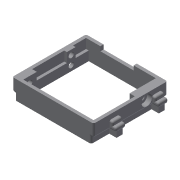
# Autodesk Inventor part: HDB Support
Saved by Autodesk Inventor 2017 (Build 210142000, 142)
## iProperties
Created: 2015-03-18
Part Number: HDB Support
Material: Generic
Document SubType Name: Modeling
Designer: PC-fabtotum
Density: 1 g/cm^3
Appearance: Default
RuleStatus: InUse
BeforeDocSave0: Spessore
Author: PC-fabtotum
Autodesk Inventor part; units mm, degrees
note: some values were not read from the file. Chosen so that the rebuilt part matches the saved one: second side of "Extrusion1".
ref_plane "Work Plane1" through (0, 0, -8.25) normal (0, 0, 1) x (1, 0, 0)
sketch "Sketch1" plane through (0, 0, -8.25) normal (0, 0, 1) x (1, 0, 0)
  line L0 (-37.1615, 17.9395) -> (9.3315, 17.9395)
  line L1 (9.3315, 17.9395) -> (9.3315, -24.2572)
  line L2 (9.3315, -24.2572) -> (-37.1615, -24.2572)
  line L3 (-37.1615, -24.2572) -> (-37.1615, 17.9395)
  point P0 (0, 0)
  constraints: 8 end point, 3 horizontal, 2 parallel, 2 vertical, 1 perpendicular, 1 other
extrude "Extrusion1" add sketch "Sketch1" along normal blind 7.25
sketch "Sketch2" plane through (0, 0, -8.25) normal (0, 0, 1) x (1, 0, 0)
  line L0 (13.1261, 14.7262) -> (3.5753, 14.7262)
  line L1 (3.5753, 14.7262) -> (3.5753, 9.2758)
  line L2 (3.5753, 9.2758) -> (13.1261, 9.2758)
  line L3 (13.1261, 9.2758) -> (13.1261, 14.7262)
  line L4 (13.1261, -9.4662) -> (3.7861, -9.4662)
  line L5 (3.7861, -9.4662) -> (3.7861, -15.116)
  line L6 (3.7861, -15.116) -> (13.1261, -15.116)
  line L7 (13.1261, -15.116) -> (13.1261, -9.4662)
  line L8 (-40.7637, 14.7262) -> (-33.7354, 14.7262)
  line L9 (-33.7354, 14.7262) -> (-33.7354, 9.2758)
  line L10 (-33.7354, 9.2758) -> (-40.7637, 9.2758)
  line L11 (-40.7637, 9.2758) -> (-40.7637, 14.7262)
  line L12 (-40.7637, -9.3156) -> (-33.2967, -9.3156)
  line L13 (-33.2967, -9.3156) -> (-33.2967, -15.116)
  line L14 (-33.2967, -15.116) -> (-40.7637, -15.116)
  line L15 (-40.7637, -15.116) -> (-40.7637, -9.3156)
  point P0 (0, 0)
  constraints: 32 end point, 11 horizontal, 8 parallel, 8 vertical, 5 point on line, 4 perpendicular, 17 other
extrude "Extrusion2" add sketch "Sketch2" along normal blind 2.5
sketch "Sketch3" plane through (0, 0, -5.75) normal (0, 0, 1) x (1, 0, 0)
  line L0 (9.3315, 9.2758) -> (13.1261, 9.2758) projected
  line L1 (11.304, 9.2758) -> (9.3315, 9.2758)
  line L2 (9.3315, 9.2758) -> (9.3315, 14.7262)
  line L3 (9.3315, 14.7262) -> (11.304, 14.7262)
  line L4 (11.304, 14.7262) -> (11.304, 9.2758)
  line L5 (9.3315, -24.2572) -> (9.3315, 17.9395) projected
  line L6 (13.1261, -9.4662) -> (9.3315, -9.4662) projected
  line L7 (11.304, -9.4662) -> (9.3315, -9.4662)
  line L8 (9.3315, -9.4662) -> (9.3315, -15.116)
  line L9 (9.3315, -15.116) -> (11.304, -15.116)
  line L10 (11.304, -15.116) -> (11.304, -9.4662)
  line L11 (-37.1615, -15.116) -> (-38.9272, -15.116)
  line L12 (-38.9272, -15.116) -> (-38.9272, -9.3156)
  line L13 (-38.9272, -9.3156) -> (-37.1615, -9.3156)
  line L14 (-37.1615, -9.3156) -> (-37.1615, -15.116)
  line L15 (-37.1615, 14.7262) -> (-40.7637, 14.7262) projected
  line L16 (-38.9272, 14.7262) -> (-37.1615, 14.7262)
  line L17 (-37.1615, 14.7262) -> (-37.1615, 9.2758)
  line L18 (-37.1615, 9.2758) -> (-38.9272, 9.2758)
  line L19 (-38.9272, 9.2758) -> (-38.9272, 14.7262)
  line L20 (13.1261, 14.7262) -> (9.3315, 14.7262) projected
  line L21 (-37.1615, -9.3156) -> (-40.7637, -9.3156) projected
  point P0 (0, 0)
  constraints: 32 end point, 8 parallel, 5 collinear, 4 horizontal, 4 perpendicular, 3 point on line, 2 vertical
extrude "Extrusion3" add sketch "Sketch3" along normal blind 2
sketch "Sketch4" plane through (0, 0, -8.25) normal (0, 0, -1) x (-1, 0, 0)
  line L0 (-9.3315, -24.2572) -> (37.1615, -24.2572) projected
  line L1 (37.1615, 17.9395) -> (-9.3315, 17.9395) projected
  line L2 (-7.9441, -24.2572) -> (35.6472, -24.2572)
  line L3 (35.6472, -24.2572) -> (35.6472, 17.9395)
  line L4 (35.6472, 17.9395) -> (-7.9441, 17.9395)
  line L5 (-7.9441, 17.9395) -> (-7.9441, -24.2572)
  point P0 (0, 0)
  constraints: 8 end point, 2 parallel, 2 point on line, 1 horizontal, 1 perpendicular
extrude "Extrusion4" add sketch "Sketch4" along normal blind 3.5
shell "Shell1" thickness 1.8 removed faces 1 at (-21.6638, -10.1916, -1)
sketch "Sketch5" plane through (-33.8472, -22.4572, -9.95) normal (0, 0, 1) x (1, 0, 0)
  line L0 (41.3787, 38.5966) -> (41.3787, 0) construction
  line L1 (41.3787, 23.5966) -> (38.3787, 23.5966)
  line L2 (38.3787, 23.5966) -> (38.3787, 38.5966)
  line L3 (38.3787, 38.5966) -> (41.3787, 38.5966)
  line L4 (41.3787, 23.5966) -> (41.3787, 38.5966)
  line L5 (-1.8, -1.0089) -> (1.1787, -1.0089)
  line L6 (1.1787, -1.0089) -> (1.1787, 7.7162)
  line L7 (1.1787, 7.7162) -> (-1.8, 7.7162)
  line L8 (-1.8, 7.7162) -> (-1.8, -1.0089)
  line L9 (-1.8, -1.8) -> (-1.8, 40.3966) projected
  line L10 (0, 0) -> (0, 38.5966) projected
  line L11 (41.3787, 33.5329) -> (41.3787, 11.191) projected
  line L12 (0, 38.5966) -> (39.9913, 38.5966) projected
  point P0 (33.8472, 22.4572)
  dimension "d69" = 37.2
  dimension "d70" = 3
  dimension "d71" = 15
  constraints: 16 end point, 3 collinear, 3 perpendicular, 2 horizontal, 2 parallel, 2 point on line
  measures "d69" distance between parallel lines of L6 L2
  measures "d70" distance between parallel lines of L2 L11
  measures "d71" distance of L1.end L2.end
extrude "Extrusion5" add sketch "Sketch5" along normal up to surface (8.95 mm away)
sketch "Sketch6" plane through (-37.1615, -24.2572, -1) normal (-1, 0, 0) x (0, 0, 1)
  point P0 (1, 24.2572)
  point P1 (-3.6337, 5.4847)
hole "Hole1" at (-37.1615, -18.7725, -4.6337) direction (1, 0, 0) diameter 3 depth 8 tip angle 118 counterbore diameter 6 counterbore depth 2.7
sketch "Sketch7" plane through (9.3315, -24.2572, -1) normal (1, 0, 0) x (0, 0, -1)
  point P0 (-1, 24.2572)
  point P1 (3.6353, 30.4382)
hole "Hole2" at (9.3315, 6.181, -4.6353) direction (-1, 0, 0) diameter 3 depth 8 tip angle 118 counterbore diameter 6 counterbore depth 2.7
sketch "Sketch8" plane through (-33.8472, 16.1395, -9.95) normal (0, 0, 1) x (1, 0, 0)
  line L0 (1.1787, -38.5966) -> (3.957, -38.5966)
  line L1 (3.957, -38.5966) -> (3.957, -39.3714)
  line L2 (3.957, -39.3714) -> (1.1787, -39.3714)
  line L3 (1.1787, -39.3714) -> (1.1787, -38.5966)
  circle A0 centre (30.4917, -32.0966) radius 7.5
  line L4 (30.4917, -32.0966) -> (30.4917, -39.5966) construction
  line L5 (-3.3143, -40.3966) -> (43.1787, -40.3966) projected
  line L6 (39.9913, -38.5966) -> (39.9913, -15) projected
  point P0 (33.8472, -16.1395)
  dimension "d51" = 15
  dimension "d50" = 0.8
  dimension "d52" = 9.4996
  constraints: 10 end point, 2 parallel, 1 horizontal, 1 perpendicular, 1 vertical, 1 vertical alignment, 2 other
  measures "d50" distance from line of L5 L4.end
  measures "d52" distance between parallel lines of L6 L4
extrude "Extrusion6" [suppressed]
sketch "Sketch9" plane through (-33.8472, 16.1395, -9.95) normal (0, 0, 1) x (1, 0, 0)
  line L0 (39.9913, -38.5966) -> (1.1787, -38.5966) construction
  line L1 (6.3811, -38.5966) -> (19.879, -38.5966)
  line L2 (19.879, -38.5966) -> (19.879, -22.0157)
  line L3 (19.879, -22.0157) -> (6.3811, -22.0157)
  line L4 (6.3811, -22.0157) -> (6.3811, -38.5966)
  line L5 (0, 0) -> (38.3787, 0) construction
  line L6 (33.1556, 0) -> (28.7955, 0)
  line L7 (28.7955, 0) -> (28.7955, -12.1404)
  line L8 (28.7955, -12.1404) -> (33.1556, -12.1404)
  line L9 (33.1556, -12.1404) -> (33.1556, 0)
  point P0 (33.8472, -16.1395)
  point P1 (26.0223, -38.1966)
  point P2 (3.6113, -38.1966)
  point P3 (39.9913, 0)
  constraints: 16 end point, 4 parallel, 2 horizontal, 2 perpendicular, 1 point on line, 2 other
extrude "Extrusion7" [suppressed]
sketch "Sketch10" plane through (-33.8472, -14.741, -9.95) normal (0, 0, 1) x (1, 0, 0)
  arc A0 (2.5514, 21.9404) -> (28.5514, 21.9404) centre (15.5514, 21.9404) ccw
  line L0 (28.5514, 21.9404) -> (28.5514, 32.6805)
  line L1 (28.5514, 32.6805) -> (2.5514, 32.6805)
  line L2 (2.5514, 32.6805) -> (2.5514, 21.9404)
  line L3 (43.1787, 32.6805) -> (-3.3143, 32.6805) projected
  line L4 (15.5514, 21.9404) -> (15.5514, 32.6805)
  line L5 (-1.8, 32.6805) -> (41.7913, 32.6805) projected
  line L6 (0, 30.8805) -> (0, 0) projected
  point P0 (33.8472, 14.741)
  dimension "d32" = 13
  dimension "d53" = 10.7401
  dimension "d54" = 15.5513
  constraints: 8 end point, 2 point on circle, 2 tangent, 1 centre point, 1 collinear, 1 parallel, 1 perpendicular, 1 point on line, 1 vertical
  measures "d32" radius of A0
  measures "d53" distance of L4.start L4.end
  measures "d54" distance between parallel lines of L6 L4
extrude "Extrusion8" [suppressed]
shell "Shell2" [suppressed]
fillet "Fillet1" [suppressed]
fillet "Fillet3" radius 1 70 edges at (-39.8455, -15.116, -5.75) (-40.7637, -15.116, -7) (-40.7637, -12.2158, -5.75) (-39.8455, -9.3156, -5.75) (-40.7637, -9.3156, -7) (-38.9272, -15.116, -4.75) (-38.9272, -9.3156, -4.75) (-38.9272, -12.2158, -3.75) (-38.0444, -9.3156, -3.75) (-38.0444, -15.116, -3.75) (-38.9626, -15.116, -8.25) (-40.7637, -12.2158, -8.25) (-38.9626, -9.3156, -8.25) (-37.1615, -19.6866, -8.25) (-36.4043, -24.2572, -8.25) (-35.6472, -24.2572, -10) (-37.1615, -24.2572, -4.625) (-40.7637, 9.2758, -7) (-39.8455, 9.2758, -5.75) (-39.8455, 14.7262, -5.75) (-40.7637, 12.001, -5.75) (-40.7637, 14.7262, -7) (-40.7637, 12.001, -8.25) (-38.9626, 9.2758, -8.25) (-38.9626, 14.7262, -8.25) (-38.9272, 14.7262, -4.75) (-38.9272, 9.2758, -4.75) (-38.0444, 9.2758, -3.75) (-38.9272, 12.001, -3.75) (-38.0444, 14.7262, -3.75) (-37.1615, -0.0199, -8.25) (-37.1615, 16.3328, -8.25) (-37.1615, 17.9395, -4.625) (-35.6472, 17.9395, -10) (-36.4043, 17.9395, -8.25) (13.1261, -12.2911, -8.25) (11.2288, -15.116, -8.25) (13.1261, -15.116, -7) (13.1261, -9.4662, -7) (13.1261, -12.2911, -5.75) (12.215, -9.4662, -5.75) (12.215, -15.116, -5.75) (10.3178, -15.116, -3.75) (11.304, -12.2911, -3.75) (11.304, -15.116, -4.75) (11.304, -9.4662, -4.75) (10.3178, -9.4662, -3.75) (9.3315, -19.6866, -8.25) (9.3315, -0.0952, -8.25) (7.9441, -24.2572, -10) (8.6378, -24.2572, -8.25) (9.3315, -24.2572, -4.625) (13.1261, 14.7262, -7) (13.1261, 9.2758, -7) (13.1261, 12.001, -5.75) (12.215, 14.7262, -5.75) (12.215, 9.2758, -5.75) (13.1261, 12.001, -8.25) (11.2288, 14.7262, -8.25) (11.2288, 9.2758, -8.25) (11.304, 9.2758, -4.75) (11.304, 12.001, -3.75) (10.3178, 9.2758, -3.75) (10.3178, 14.7262, -3.75) (11.304, 14.7262, -4.75) (9.3315, 16.3328, -8.25) (8.6378, 17.9395, -8.25) (9.3315, 17.9395, -4.625) (7.9441, 17.9395, -10) (11.2288, -9.4662, -8.25)
sketch "Sketch12" plane through (0, 0, -11.75) normal (0, 0, -1) x (-1, 0, 0)
  circle A0 centre (3.536, -9.9787) radius 7.2457
  point P0 (0, 0)
  constraints: 1 centre point
extrude "Extrusion9" [suppressed]
fillet "Fillet4" radius 0.5 3 edges at (-35.3543, -23.9643, -7.9571) (-35.3543, 17.6466, -7.9571) (-35.6472, -3.1588, -8.25)
sketch "Sketch13" plane through (0, 0, -8.25) normal (0, 0, -1) x (-1, 0, 0)
  line L0 (-12.1261, 13.7262) -> (-12.1261, 10.2758)
  line L1 (-12.1261, 13.7262) -> (-12.1261, 10.2758) projected
  line L2 (-12.1261, 10.2758) -> (-7.9441, 10.2758)
  line L3 (-12.1261, 13.7262) -> (-7.9441, 13.7262)
  line L4 (-7.9441, 13.2762) -> (-11.6761, 13.2762)
  line L5 (-11.6761, 13.2762) -> (-11.6761, 10.7258)
  line L6 (-11.6761, 10.7258) -> (-7.9441, 10.7258)
  line L7 (-7.9441, 13.7262) -> (-7.9441, 13.2762)
  line L8 (-7.9441, -23.2572) -> (-7.9441, 16.9395) projected
  line L9 (-7.9441, 10.7258) -> (-7.9441, 10.2758)
  point P0 (0, 0)
  dimension "d46" = 0.45
  constraints: 16 end point, 3 collinear, 2 parallel, 2 perpendicular, 2 other
  measures "d46" distance between parallel lines of L2 L6
extrude "Extrusion10" add sketch "Sketch13" along normal up to surface (3.5 mm away) contours L3 L7 L4 L5 L6 L8 L2 L0
ref_plane "Work Plane2" through (9.3315, -0.0952, -7.25) normal (0, 1, 0) x (1, 0, 0)
ref_plane "Work Plane3" through (-13.8515, -23.2572, -8.25) normal (1, 0, 0) x (0, 0, -1)
mirror "Mirror1" about plane through (-13.8515, -23.2572, -8.25) normal (1, 0, 0) of "Extrusion10"
mirror "Mirror2" about plane through (9.3315, -0.0952, -7.25) normal (0, 1, 0) of "Extrusion10", "Mirror1"
sketch "Schizzo15" plane through (-33.8472, 16.1395, -9.95) normal (0, 0, 1) x (1, 0, 0)
  line L0 (39.9913, -15) -> (39.9913, -38.5966) projected
  line L1 (0, 0) -> (38.3787, 0) projected
  line L2 (0, -30.8805) -> (0, 0) projected
  line L3 (39.9913, -38.5966) -> (1.1787, -38.5966) projected
  line L4 (38.3787, -15) -> (38.3787, 0) projected
  line L5 (0, -30.8805) -> (1.1787, -30.8805) projected
  line L6 (1.1787, -30.8805) -> (1.1787, -38.5966) projected
  line L7 (39.9913, -15) -> (38.3787, -15) projected
  point P0 (33.8472, -16.1395)
extrude "Estrusione12" cut sketch "Schizzo15" against normal blind 10
sketch "Schizzo18" plane through (-35.3615, -11.1156, -6.45) normal (1, 0, 0) x (0, 0, -1)
  line L0 (0, 14.7551) -> (-5.45, 14.7551)
  line L1 (-5.45, 14.7551) -> (-5.45, 19.7551)
  line L2 (-5.45, 19.7551) -> (0, 19.7551)
  line L3 (0, 19.7551) -> (0, 14.7551)
  line L4 (-5.45, -3.6254) -> (-5.45, 27.2551) projected
  line L5 (0, 0) -> (0, 22.1914) projected
  line L6 (0, 27.2551) -> (-5.45, 27.2551) projected
  point P0 (-6.45, 11.1156)
  dimension "d77" = 5
  dimension "d78" = 7.5
  constraints: 8 end point, 2 collinear, 2 parallel, 1 horizontal, 1 perpendicular
  measures "d77" distance between parallel lines of L2 L0
  measures "d78" distance between parallel lines of L2 L6
extrude "Estrusione15" add sketch "Schizzo18" along normal up to surface (1.5143 mm away)
sketch "Schizzo16" plane through (-33.8472, 16.1395, -6.45) normal (1, 0, 0) x (0, 0, -1)
  circle A0 centre (2.3, -10) radius 1.5
  line L0 (0, 0) -> (5.3, 0) projected
  line L1 (5.3, 0) -> (5.3, -38.5966) projected
  line L2 (2.3, -10) -> (-2.7, -10) construction
  circle A1 centre (-2.7, -10) radius 1.5
  point P0 (-6.45, -16.1395)
  point P1 (5.3, -30.8805)
  dimension "d62" = 3
  dimension "d63" = 10
  dimension "d64" = 3
  dimension "d65" = 5
  dimension "d66" = 3
  constraints: 2 centre point, 2 end point, 1 coincident, 1 horizontal
  measures "d62" diameter of A0
  measures "d63" distance from line of L0 L2.start
  measures "d64" distance from line of L2.start L1
  measures "d65" distance of L2.start L2.end
  measures "d66" diameter of A1
extrude "Estrusione13" cut sketch "Schizzo16" against normal blind 10
sketch "Schizzo19" plane through (7.5315, -22.4572, -6.45) normal (-1, 0, 0) x (0, 0, 1)
  line L0 (5.45, 23.5966) -> (0, 23.5966) projected
  line L1 (0, 23.5966) -> (0, 11.191) projected
  line L2 (0.9, 11.191) -> (0, 11.191) projected
  line L3 (0.9, 9.1412) -> (0.9, 11.191) projected
  line L4 (0, 9.1412) -> (0.9, 9.1412) projected
  line L5 (0, 9.1412) -> (0, 0) projected
  line L6 (0, 0) -> (5.45, 0) projected
  line L7 (5.45, 23.5966) -> (5.45, 0) projected
  line L8 (0, 11.191) -> (0, 9.1412)
  point P0 (6.45, 22.4572)
  constraints: 2 end point, 1 collinear
extrude "Estrusione16" add sketch "Schizzo19" against normal up to surface (1.9725 mm away) contours L2 L3 L4 L8
sketch "Schizzo20" plane through (-35.3615, -13.316, -5.55) normal (1, 0, 0) x (0, 0, -1)
  line L0 (0.9, 16.9555) -> (-4.55, 16.9555) projected
  line L1 (-4.55, -1.425) -> (-4.55, 16.9555) projected
  line L2 (-4.55, -1.425) -> (0.9, -1.425) projected
  line L3 (0.9, -1.425) -> (0.9, 0) projected
  line L4 (0, 0) -> (0.9, 0) projected
  line L5 (0, 2.2004) -> (0, 0) projected
  line L6 (0.9, 2.2004) -> (0, 2.2004) projected
  line L7 (0.9, 2.2004) -> (0.9, 16.9555) projected
  line L8 (1.7, 28.0422) -> (1.7, 27.0422) projected
  line L9 (-4.55, 21.9555) -> (0.9, 21.9555) projected
  line L10 (0.9, 21.9555) -> (0.9, 24.3918) projected
  line L11 (0, 24.3918) -> (0.9, 24.3918) projected
  line L12 (0, 26.2422) -> (0, 24.3918) projected
  line L13 (0.9, 26.2422) -> (0, 26.2422) projected
  line L14 (0.9, 26.2422) -> (0.9, 29.4555) projected
  line L15 (0.9, 29.4555) -> (-4.55, 29.4555) projected
  line L16 (-4.55, 21.9555) -> (-4.55, 29.4555) projected
  line L17 (0.9, 26.2422) -> (0.9, 24.3918)
  line L18 (0.9, 0) -> (0.9, 2.2004)
  point P0 (-5.55, 13.316)
  constraints: 4 end point, 1 collinear, 1 vertical
extrude "Estrusione17" add sketch "Schizzo20" against normal up to next contours L18 L4 L5 L6 | L11 L12 L13 L17
sketch "Schizzo17" plane through (-36.1615, 17.9395, -1) normal (0, 1, 0) x (1, 0, 0)
  line L0 (44.493, 0) -> (0, 0) projected
  line L1 (9, 0) -> (28, 0)
  line L2 (28, 0) -> (28, 2.5)
  line L3 (28, 2.5) -> (9, 2.5)
  line L4 (9, 2.5) -> (9, 0)
  line L5 (-1, 6.25) -> (-1, 0) projected
  point P0 (36.1615, -1)
  dimension "d72" = 10
  dimension "d73" = 19
  dimension "d74" = 2.5
  constraints: 8 end point, 2 parallel, 1 horizontal, 1 perpendicular, 1 point on line
  measures "d72" distance between parallel lines of L5 L4
  measures "d73" distance of L2.end L3.end
  measures "d74" distance of L1.end L2.end
extrude "Estrusione14" cut sketch "Schizzo17" against normal blind 10
sketch "Sketch14" plane through (-5.0958, 7.1994, -9.75) normal (-1, 0, 0) x (0, 0, 1)
  line L0 (8.75, 10.7401) -> (8.75, 8.7401) construction
  line L1 (-2, 10.7401) -> (8.75, 10.7401) projected
  line L2 (-2, 0) -> (-2, 10.7401) construction
  line L3 (-2, 10.7401) -> (-2, 9.9401)
  line L4 (-2, 9.9401) -> (8.75, 9.9401)
  line L5 (8.75, 9.9401) -> (8.75, 10.7401)
  point P0 (9.75, -7.1994)
  point P1 (0, 8.7401)
  dimension "d57" = 0.8
  constraints: 6 end point, 2 point on line, 1 collinear, 1 horizontal
  measures "d57" distance between parallel lines of L1 L4
extrude "Extrusion11" [suppressed]
fillet "Fillet5" [suppressed]
fillet "Fillet6" [suppressed]
body "Solid1"
